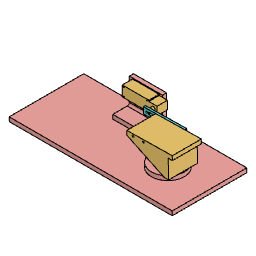
Sicherheitsabdeckung (Autodesk Fusion 360 design; units mm, degrees)
Autodesk Fusion 360 part; units mm, degrees
sketch "Sketch1" plane through (0, 0, 0) normal (0, 0, 1) x (1, 0, 0) in component "Schalter"
  circle A0 centre (4, 23) radius 1.5
  circle A1 centre (4, 2) radius 1.5
  circle A2 centre (60, 23) radius 1.5
  circle A3 centre (60, 2) radius 1.5
  circle A4 centre (74, 12.5) radius 5
  line L0 (0, 0) -> (0, 25)
  line L1 (0, 25) -> (64, 25)
  line L2 (64, 25) -> (64, 22.5)
  line L3 (64, 22.5) -> (84, 22.5)
  line L4 (84, 22.5) -> (84, 2.5)
  line L5 (84, 2.5) -> (64, 2.5)
  line L6 (64, 2.5) -> (64, 0)
  line L7 (64, 0) -> (0, 0)
  dimension "d23" = 25
  dimension "d25" = 64
  dimension "d26" = 20
  dimension "d27" = 20
  dimension "d28" = 3
  dimension "d29" = 10
  dimension "d30" = 10
  dimension "d31" = 10
  dimension "d81" = 21
  dimension "d82" = 56
  dimension "d83" = 2
  constraint coincident L0.start L7.end
  constraint vertical L0
  constraint perpendicular L1 L2
  constraint perpendicular L3 L4
  constraint horizontal L5
  constraint perpendicular L3 L6
  constraint perpendicular L2 L3
  constraint perpendicular L0 L1
  constraint horizontal L7
  constraint collinear L2 L6
  constraint equal A0 A2
  constraint equal A2 A3
  constraint equal A1 A3
  constraint equal L2 L6
  constraint vertical A2.centre A3.centre
  constraint horizontal A1.centre A3.centre
  constraint vertical A0.centre A1.centre
  constraint horizontal A0.centre A2.centre
  measures "d23" distance of L0.start L0.end
  measures "d25" distance of L6.end L0.start
  measures "d26" distance of L2.end L3.end
  measures "d27" distance of L3.end L4.end
  measures "d28" diameter of A2
  measures "d29" diameter of A4
  measures "d30" vertical distance of A4.centre L2.end
  measures "d31" horizontal distance of A4.centre L1.end
  measures "d81" vertical distance of A0.centre A1.centre
  measures "d82" horizontal distance of A0.centre A2.centre
  measures "d83" distance of A0.centre L1
extrude "Extrude1" add sketch "Sketch1" along normal blind 25 makes body 1 in component "Schalter"
sketch "Sketch1 (2)" plane through (0, 0, 0) normal (0, 0, 1) x (1, 0, 0) in component "Hebel"
  line L0 (0, 0) -> (100, 0)
  line L1 (100, 0) -> (100, 15)
  line L2 (100, 15) -> (0, 15)
  line L3 (0, 15) -> (0, 0)
  line L4 (12, 5) -> (75, 5)
  line L5 (75, 5) -> (75, 10)
  line L6 (75, 10) -> (12, 10)
  line L7 (12, 10) -> (12, 5)
  circle A0 centre (8, 7.5) radius 2
  dimension "d32" = 100
  dimension "d33" = 15
  dimension "d34" = 7.5
  constraint horizontal L0
  constraint vertical L1
  constraint horizontal L2
  constraint vertical L3
  constraint coincident L0.start L3.end
  constraint horizontal L4
  constraint vertical L5
  constraint horizontal L6
  constraint vertical L7
  measures "d32" distance of L1.end L2.end
  measures "d33" distance of L0.start L2.end
  measures "d34" distance of L0 A0.centre
extrude "Extrude1'" add sketch "Sketch1 (2)" along normal blind 5 separate body makes body 2 in component "Hebel"
sketch "Sketch1 (3)" plane through (0, 0, 0) normal (0, 0, 1) x (1, 0, 0) in component "Maschinenoberseite"
  line L0 (-86.8904, 53.8556) -> (306.9807, 53.8556)
  line L1 (306.9807, 53.8556) -> (306.9807, -126.4802)
  line L2 (306.9807, -126.4802) -> (-86.8904, -126.4802)
  line L3 (-86.8904, -126.4802) -> (-86.8904, 53.8556)
  circle A0 centre (210, -40) radius 40
  circle A1 centre (210, -40) radius 15
  circle A2 centre (210, -40) radius 11
  dimension "d71" = 80
  dimension "d72" = 30
  dimension "d73" = 22
  constraint horizontal L0
  constraint vertical L1
  constraint horizontal L2
  constraint vertical L3
  constraint concentric A0 A1
  constraint concentric A1 A2
  measures "d71" diameter of A0
  measures "d72" diameter of A1
  measures "d73" diameter of A2
extrude "Extrude1''" add sketch "Sketch1 (3)" against normal blind 10 separate body contours L0 L1 L2 L3 | A0 | A1 | A2 makes body 3 in component "Maschinenoberseite"
extrude "Extrude2" add sketch "Sketch1 (3)" along normal blind 10 contours A0 | A1 | A2 bodies 3 in component "Maschinenoberseite"
extrude "Extrude3" add sketch "Sketch1 (3)" along normal blind 40 contours A1 | A2 bodies 3 in component "Maschinenoberseite"
extrude "Extrude4" add sketch "Sketch1 (3)" along normal blind 50 contours A2 bodies 3 in component "Maschinenoberseite"
sketch "Sketch1 (4)" plane through (0, 0, 0) normal (0, 1, 0) x (1, 0, 0) in component "Deckel"
  line L0 (245, -60) -> (345, -60)
  line L1 (345, -60) -> (345, -5)
  line L2 (345, -5) -> (245, -5)
  line L3 (245, -5) -> (245, -60)
  line L4 (245, -50) -> (335, -50)
  line L5 (335, -50) -> (335, -5)
  line L6 (335, -5) -> (245, -5)
  line L7 (245, -5) -> (245, -50)
  circle A0 centre (260, -55) radius 2
  circle A1 centre (285, -55) radius 2
  line L8 (245, -50) -> (335, -5)
  line L9 (345, -60) -> (355, -60)
  line L10 (355, -60) -> (355, -50)
  line L11 (355, -50) -> (345, -50)
  dimension "d74" = 4
  dimension "d75" = 4
  dimension "d90" = 55
  dimension "d91" = 90
  dimension "d92" = 100
  dimension "d93" = 10
  dimension "d94" = 15
  dimension "d95" = 25
  dimension "d96" = 5
  constraint horizontal L0
  constraint vertical L1
  constraint horizontal L2
  constraint vertical L3
  constraint horizontal L4
  constraint vertical L5
  constraint horizontal L6
  constraint vertical L7
  constraint coincident L2 L5.end
  constraint coincident L3 L4.start
  constraint horizontal A0.centre A1.centre
  constraint perpendicular L1 L9
  constraint perpendicular L9 L10
  constraint coincident L1 L11.end
  constraint perpendicular L1 L11
  measures "d74" diameter of A0
  measures "d75" diameter of A1
  measures "d90" distance of L0.start L2.end
  measures "d91" distance of L5.end L2.end
  measures "d92" distance of L1.end L2.end
  measures "d93" distance of L0 L4
  measures "d94" distance of L3 A0.centre
  measures "d95" distance of A0.centre A1.centre
  measures "d96" distance of L0 A0.centre
extrude "Extrude1'''" add sketch "Sketch1 (4)" against normal blind 70 separate body contours L0 L1 L2 L3 L4 L5 | L1 L9 L10 L11 makes body 4 in component "Deckel"
extrude "Extrude3'" add sketch "Sketch1 (4)" against normal blind 5 contours L4 L5 L8 bodies 4 in component "Deckel"
extrude "Extrude4'" add sketch "Sketch1 (4)" along normal blind -70 and the other way blind 65 contours L4 L5 L8 bodies 4 in component "Deckel"
sketch "Sketch2" plane through (0, 0, 0) normal (0, 0, 1) x (1, 0, 0) in component "Haltewinkel"
  line L0 (0, 0) -> (80, 0)
  line L1 (80, 0) -> (80, 50)
  line L2 (80, 50) -> (0, 50)
  line L3 (0, 50) -> (0, 0)
  line L4 (0, 40) -> (80, 40)
  constraint horizontal L0
  constraint vertical L1
  constraint horizontal L2
  constraint vertical L3
  constraint coincident L0.start L3.end
  constraint coincident L3 L4.start
  constraint coincident L1 L4.end
  constraint perpendicular L1 L4
extrude "Extrude2'" add sketch "Sketch2" against normal blind 10 separate body makes body 5 in component "Haltewinkel"
extrude "Extrude3''" add sketch "Sketch2" along normal blind 60 contours L1 L2 L3 L4 bodies 5 in component "Haltewinkel"
sketch "Sketch3" plane through (0, 40, 0) normal (0, -1, 0) x (1, 0, 0) in component "Haltewinkel"
  line L0 (0, 0) -> (80, 0)
  line L1 (80, 0) -> (80, 60)
  line L2 (80, 60) -> (0, 60)
  line L3 (0, 60) -> (0, 0)
  circle A0 centre (12, 55) radius 2.25
  circle A1 centre (12, 34) radius 2.25
  circle A2 centre (68, 55) radius 2.25
  circle A3 centre (68, 34) radius 2.25
  dimension "d62" = 4.5
  dimension "d79" = 56
  dimension "d80" = 21
  dimension "d97" = 12
  dimension "d98" = 5
  constraint equal A2 A3
  constraint equal A0 A2
  constraint equal A0 A1
  constraint horizontal A0.centre A2.centre
  constraint horizontal A1.centre A3.centre
  constraint vertical A0.centre A1.centre
  constraint vertical A2.centre A3.centre
  measures "d62" diameter of A0
  measures "d79" distance of A0.centre A2.centre
  measures "d80" distance of A0.centre A1.centre
  measures "d97" distance of L3 A0.centre
  measures "d98" distance of L2 A0.centre
fillet "Fillet1" radius 5 1 edges at (40, 40, 0) on bodies 5 in component "Haltewinkel"
extrude "Extrude4''" cut sketch "Sketch3" against normal blind 10 contours A0 | A1 | A2 | A3 bodies 5 in component "Haltewinkel"
component "Haltewinkel" placed x (1, 0, 0) y (0, 1, 0) z (0, 0, 1) at (43.1096, -6.1444, 10)
component "Schalter" placed x (1, 0, 0) y (0, 0, 1) z (0, -1, 0) at (51.1096, 33.8556, 43)
component "Hebel" placed x (1, 0, 0) y (0, 0, 1) z (0, -1, 0) at (117.1096, -1.1444, 48)
component "Maschinenoberseite" placed x (1, 0, 0) y (0, 1, 0) z (0, 0, 1) at (0, 0, 0)
component "Deckel" placed x (1, 0, 0) y (0, 1, 0) z (0, 0, 1) at (-97.8904, -6.1444, 3)
equation "d34 = d33 / 2"
equation "d74 = d75"
